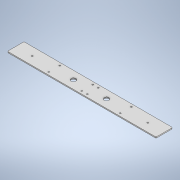
# Autodesk Inventor part: sidePanel v1
Saved by Autodesk Inventor 2020 (Build 240168000, 168)
## iProperties
Created: 2019-11-14
Part Number: sidePanel v1
Material: Generic
Document SubType Name: Modeling
Designer: xj82b
Density: 1 g/cm^3
Appearance: Default
Author: xj82b
Autodesk Inventor part; units mm, degrees
ref_plane "YZ Plane" through (0, 0, 0) normal (1, 0, 0) x (0, 1, 0)
ref_plane "XZ Plane" through (0, 0, 0) normal (0, 1, 0) x (-1, 0, 0)
ref_plane "XY Plane" through (0, 0, 0) normal (0, 0, 1) x (1, 0, 0)
sketch "Sketch1" plane through (0, 0, 0) normal (0, 1, 0) x (-1, 0, 0)
  line L0 (-2, 0) -> (-430, 0)
  line L1 (-432, -2) -> (-432, -46)
  line L2 (-430, -48) -> (-2, -48)
  line L3 (0, -46) -> (0, -2)
  circle A0 centre (-112, -40) radius 2
  circle A1 centre (-112, -8) radius 2
  circle A2 centre (-208, -40) radius 2
  circle A3 centre (-224, -40) radius 2
  circle A4 centre (-224, -8) radius 2
  circle A5 centre (-208, -8) radius 2
  circle A6 centre (-320, -40) radius 2
  circle A7 centre (-320, -8) radius 2
  circle A8 centre (-48, -24) radius 2
  circle A9 centre (-384, -24) radius 2
  circle A10 centre (-168, -24) radius 7
  circle A11 centre (-264, -24) radius 7
  arc A12 (-2, -48) -> (0, -46) centre (-2, -46) ccw
  arc A13 (0, -2) -> (-2, 0) centre (-2, -2) ccw
  arc A14 (-432, -46) -> (-430, -48) centre (-430, -46) ccw
  arc A15 (-430, 0) -> (-432, -2) centre (-430, -2) ccw
  point P0 (0, 0)
  point P1 (-432, -48)
  point P2 (-432, 0)
  point P3 (0, -48)
  point P4 (0, -24)
  point P5 (-432, -24)
  dimension "d0" = 432
  dimension "d1" = 48
  dimension "d2" = 4
  dimension "d3" = 4
  dimension "d4" = 4
  dimension "d5" = 4
  dimension "d6" = 4
  dimension "d7" = 4
  dimension "d8" = 4
  dimension "d9" = 4
  dimension "d10" = 208
  dimension "d11" = 208
  dimension "d12" = 8
  dimension "d13" = 8
  dimension "d14" = 8
  dimension "d15" = 112
  dimension "d16" = 112
  dimension "d17" = 4
  dimension "d18" = 48
  dimension "d19" = 4
  dimension "d20" = 48
  dimension "d21" = 14
  dimension "d22" = 14
  dimension "d23" = 168
  dimension "d24" = 168
  dimension "d25" = 2
  constraints: 16 centre point, 9 horizontal alignment, 8 end point, 8 point on circle, 8 point on line, 8 tangent, 4 vertical alignment, 3 equal radius, 2 midpoint, 2 parallel, 1 horizontal, 1 perpendicular
  measures "d0" distance of point (0, -48) point (-432, -48)
  measures "d1" distance of point (-432, -48) point (-432, 0)
  measures "d2" diameter of A0
  measures "d3" diameter of A1
  measures "d4" diameter of A2
  measures "d5" diameter of A3
  measures "d6" diameter of A4
  measures "d7" diameter of A5
  measures "d8" diameter of A6
  measures "d9" diameter of A7
  measures "d10" distance from line of L3 A2.centre
  measures "d11" distance from line of L1 A3.centre
  measures "d12" distance from line of L2 A2.centre
  measures "d13" distance from line of L2 A3.centre
  measures "d14" distance from line of L0 A4.centre
  measures "d15" distance from line of L3 A0.centre
  measures "d16" distance from line of L1 A6.centre
  measures "d17" diameter of A8
  measures "d18" distance from line of L3 A8.centre
  measures "d19" diameter of A9
  measures "d20" distance from line of L1 A9.centre
  measures "d21" diameter of A10
  measures "d22" diameter of A11
  measures "d23" distance from line of L1 A11.centre
  measures "d24" distance from line of L3 A10.centre
  measures "d25" radius of A12
extrude "Extrusion1" add sketch "Sketch1" along normal blind 3.175
body "Solid1"
